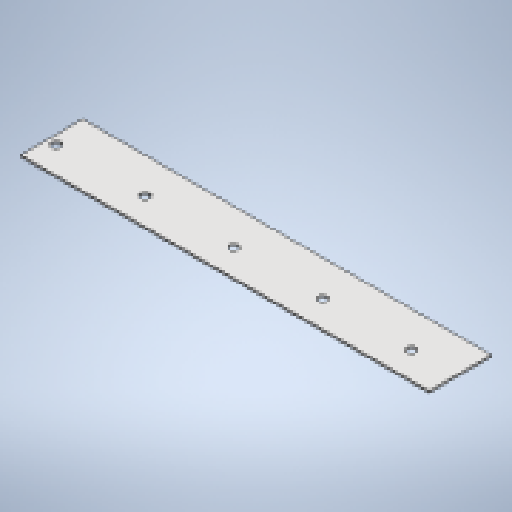
# Autodesk Inventor part: TRM 032 plate
Saved by Autodesk Inventor 2025.1 (Build 291241020, 241B)
## iProperties
Created: 2024-09-08
Part Number: TRM 032 plate
Material: Stainless Steel
Document SubType Name: Sheet Metal
Designer: pokla
Density: 8 g/cm^3
Sheet Metal Rule: AISI304 2mm Die16
Appearance: Default
Author: pokla
Autodesk Inventor part; units mm, degrees
ref_plane "YZ Plane" through (0, 0, 0) normal (1, 0, 0) x (0, 1, 0)
ref_plane "XZ Plane" through (0, 0, 0) normal (0, 1, 0) x (-1, 0, 0)
ref_plane "XY Plane" through (0, 0, 0) normal (0, 0, 1) x (1, 0, 0)
sketch "Sketch1" plane through (0, 0, 0) normal (0, 0, 1) x (1, 0, 0)
  line L0 (-230, 0) -> (230, 0)
  line L1 (230, 0) -> (230, -70)
  line L2 (230, -70) -> (-230, -70)
  line L3 (-230, -70) -> (-230, 0)
  point P0 (0, 0)
  point P1 (0, 0)
  dimension "d0" = 460
  dimension "d1" = 70
  measures "d0" distance of L0.start L0.end
  measures "d1" distance of L2.end L0.start
extrude "Plate1" add sketch "Sketch1" against normal blind 2
sketch "Sketch2" plane through (0, 0, 0) normal (0, 0, 1) x (1, 0, 0)
  line L0 (-230, -70) -> (230, -70) projected
  line L1 (230, -70) -> (230, 0) projected
  line L2 (230, 0) -> (-230, 0) projected
  line L3 (-230, 0) -> (-230, -70) projected
  circle A0 centre (180, -40) radius 5
  point P0 (0, 0)
  dimension "d3" = 10
  dimension "d4" = 50
  dimension "d5" = 30
  constraints: 1 centre point
  measures "d3" diameter of A0
  measures "d4" distance from line of L1 A0.centre
  measures "d5" distance from line of L0 A0.centre
extrude "Cut1" cut sketch "Sketch2" against normal through all contours A0
pattern_linear "Rectangular Pattern1" count 5 spacing 100 along (-1, 0, 0) of "Cut1"
equation "\"d6\" = Thickness"
equation "\"d2\" = Thickness"
equation "\"BendReliefWidth\" = Thickness"
equation "\"BendReliefDepth\" = 0.5 * Thickness"
equation "\"CornerReliefSize\" = 4 * Thickness"
equation "\"MinimumRemnant\" = 2 * Thickness"
equation "\"TransitionRadius\" = BendRadius"
equation "\"JacobiRadiusSize\" = BendRadius"
equation "\"GapSize\" = Thickness"
equation "\"Thickness\" = 2"
equation "\"BendRadius\" = 2.75"
body "Solid1"
